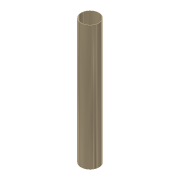
# Autodesk Inventor part: PP-11
Saved by Autodesk Inventor 2022 (Build 260148000, 148)
## iProperties
Created: 2008-09-23
Part Number: PP-11
Document SubType Name: Modeling
Designer: Mark Flayler
Mass: 2.51049 g
Surface Area: 30.5285 cm^2
Volume: 0.319401 cm^3
Density: 7.86 g/cm^3
Material: Steel, Mild
Description: SLEEVE
Appearance: Titanium - Polished
Author: Mark Flayler
Autodesk Inventor part; units mm, degrees
ref_plane "YZ Plane" through (0, 0, 0) normal (1, 0, 0) x (0, 1, 0)
ref_plane "XZ Plane" through (0, 0, 0) normal (0, 1, 0) x (-1, 0, 0)
ref_plane "XY Plane" through (0, 0, 0) normal (0, 0, 1) x (1, 0, 0)
sketch "Sketch1" plane through (0, 0, 0) normal (0, 0, 1) x (1, 0, 0)
  circle A0 centre (0, 0) radius 4.25
  circle A1 centre (0, 0) radius 4.04
  dimension "d0" = 8.5
  dimension "d1" = 8.08
  constraints: 2 centre point, 2 coincident
  measures "d0" diameter of A0
  measures "d1" diameter of A1
extrude "Extrusion1" add sketch "Sketch1" along normal blind 58.4
body "Solid1"
